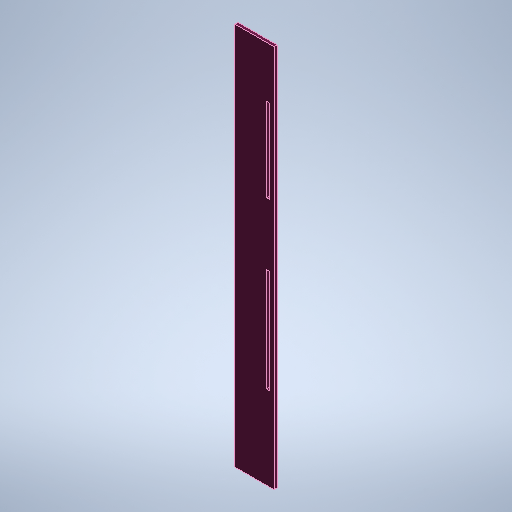
# Autodesk Inventor part: Path Side Wall
Saved by Autodesk Inventor 2025.4 (Build 294407000, 407)
## iProperties
Created: 2026-04-10
Part Number: Path Side Wall
Material: Generic
Document SubType Name: Sheet Metal
Designer: lenovo
Density: 1 g/cm^3
Sheet Metal Rule: Default_mm
Appearance: Default(1)
Author: lenovo
Autodesk Inventor part; units mm, degrees
ref_plane "YZ Plane" through (0, 0, 0) normal (1, 0, 0) x (0, 1, 0)
ref_plane "XZ Plane" through (0, 0, 0) normal (0, 1, 0) x (-1, 0, 0)
ref_plane "XY Plane" through (0, 0, 0) normal (0, 0, 1) x (1, 0, 0)
sketch "Sketch1" plane through (0, 0, 0) normal (0, 0, 1) x (1, 0, 0)
  line L0 (-19, -241) -> (19, -241)
  line L1 (19, -241) -> (19, 241)
  line L2 (19, 241) -> (-19, 241)
  line L3 (-19, 241) -> (-19, -241)
  line L4 (-19, -241) -> (19, 241) construction
  line L5 (19, -241) -> (-19, 241) construction
  line L6 (15, 191.5) -> (11.8, 191.5)
  line L7 (11.8, 191.5) -> (11.8, 110.5)
  line L8 (11.8, 110.5) -> (15, 110.5)
  line L9 (15, 110.5) -> (15, 191.5)
  line L10 (-19, 0) -> (19, 0)
  line L11 (0, 241) -> (0, -241)
  line L12 (11.8, 50) -> (15, 50)
  line L13 (15, 50) -> (15, -50)
  line L14 (15, -50) -> (11.8, -50)
  line L15 (11.8, -50) -> (11.8, 50)
  line L16 (-19, -131) -> (19, -131)
  point P0 (0, 0)
  point P1 (11.8, 0)
  point P2 (0, 0)
  dimension "d0" = 38
  dimension "d1" = 482
  dimension "d2" = 81
  dimension "d3" = 49.5
  dimension "d4" = 4
  dimension "d5" = 3.2
  dimension "d6" = 3.2
  dimension "d7" = 100
  dimension "d8" = 4
  dimension "d10" = 110
  measures "d0" distance of L2.end L1.end
  measures "d1" distance of L1.end L0.end
  measures "d2" distance of L6.end L7.end
  measures "d3" distance between parallel lines of L2 L6
  measures "d4" distance between parallel lines of L1 L9
  measures "d5" distance between parallel lines of L9 L7
  measures "d6" distance of L13.end L14.end
  measures "d7" distance of L12.end L13.end
  measures "d8" distance between parallel lines of L13 L1
  measures "d10" distance between parallel lines of L0 L16
extrude "Plate1" add sketch "Sketch1" along normal mid plane 3 contours L3 L10 L11 L16 | L11 L10 L15 L14 L13 L1 L16 | L3 L2 L11 L10 | L11 L2 L1 L10 L13 L12 L15
equation "\"d9\" = Thickness"
equation "\"BendRadius\" = Thickness"
equation "\"BendReliefWidth\" = Thickness"
equation "\"BendReliefDepth\" = 0.5 * Thickness"
equation "\"CornerReliefSize\" = 4 * Thickness"
equation "\"MinimumRemnant\" = 2 * Thickness"
equation "\"TransitionRadius\" = BendRadius"
equation "\"JacobiRadiusSize\" = BendRadius"
equation "\"GapSize\" = Thickness"
equation "\"Thickness\" = 3"
body "Solid1"
